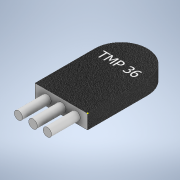
# Autodesk Inventor part: tmp 36 now
Saved by Autodesk Inventor 2021 (Build 250183000, 183)
## iProperties
Created: 2021-07-14
Part Number: tmp 36 now
Material: Generic
Document SubType Name: Modeling
Designer: Dell
Density: 1 g/cm^3
Appearance: Default
Author: Dell
Autodesk Inventor part; units mm, degrees
ref_plane "YZ Plane" through (0, 0, 0) normal (1, 0, 0) x (0, 1, 0)
ref_plane "XZ Plane" through (0, 0, 0) normal (0, 1, 0) x (-1, 0, 0)
ref_plane "XY Plane" through (0, 0, 0) normal (0, 0, 1) x (1, 0, 0)
sketch "Sketch1" plane through (0, 0, 0) normal (0, 1, 0) x (-1, 0, 0)
  line L0 (0, 0) -> (55, 0)
  line L1 (55, 0) -> (55, -90)
  line L2 (55, -90) -> (0, -90)
  line L3 (0, -90) -> (0, 0)
  dimension "d0" = 90
  dimension "d1" = 55
  constraints: 8 end point, 2 parallel, 1 horizontal, 1 perpendicular
  measures "d0" distance of L0.end L1.end
  measures "d1" distance of L1.end L2.end
extrude "Extrusion1" add sketch "Sketch1" along normal blind 15
full round fillet "Fillet1" first side at (0, 5, -30) centre faces at (-18.3333, 5, -90) second side at (-55, 5, -60)
sketch "Sketch2" plane through (-55, 0, 0) normal (0, 0, 1) x (1, 0, 0)
  circle A0 centre (12.5986, 7.0416) radius 4.3081
  circle A1 centre (27.8976, 7.0416) radius 4.5356
  circle A2 centre (42.8926, 7.0416) radius 4.3708
  point P0 (55, 0)
  constraints: 3 centre point
extrude "Extrusion2" add sketch "Sketch2" along normal blind 30
sketch "Sketch3" plane through (0, 15, 0) normal (0, 1, 0) x (1, 0, 0)
  line L0 (-48.594, 65.8616) -> (-7.6272, 65.8616) construction
  line L1 (-7.6272, 65.8616) -> (-7.6272, 56.4823) construction
  line L2 (-7.6272, 56.4823) -> (-48.594, 56.4823) construction
  line L3 (-48.594, 56.4823) -> (-48.594, 65.8616) construction
  point P0 (0, 0)
  dimension "d2" = 15
  dimension "d3" = 0
  constraints: 2 other
body "Solid1"
